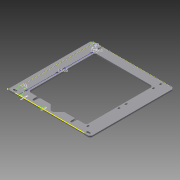
# Autodesk Inventor part: main_frame
Saved by Autodesk Inventor 2015 (Build 190159000, 159)
## iProperties
Created: 2014-12-25
Part Number: main_frame
Material: Generic
Document SubType Name: Modeling
Designer: X
Density: 1 g/cm^3
Appearance: Default
Author: X
Autodesk Inventor part; units mm, degrees
ref_plane "YZ Plane" through (0, 0, 0) normal (1, 0, 0) x (0, 1, 0)
ref_plane "XZ Plane" through (0, 0, 0) normal (0, 1, 0) x (-1, 0, 0)
ref_plane "XY Plane" through (0, 0, 0) normal (0, 0, 1) x (1, 0, 0)
sketch "Sketch1" plane through (0, 0, 0) normal (0, 0, 1) x (1, 0, 0)
  line L0 (7, 0) -> (363, 0)
  line L1 (370, 7) -> (370, 370)
  line L2 (363, 377) -> (7, 377)
  line L3 (0, 370) -> (0, 7)
  line L4 (7, 0) -> (0, 7)
  line L5 (-121.5053, 188.5) -> (511.4947, 188.5) construction
  line L6 (185, 402) -> (185, -38) construction
  line L7 (363, 0) -> (370, 7)
  line L8 (7, 377) -> (0, 370)
  line L9 (363, 377) -> (370, 370)
  point P0 (0, 0)
  point P1 (185, 377)
  point P2 (370, 188.5)
  dimension "height" = 370
  dimension "width" = 370
  dimension "Chamfer1" = 7
  dimension "Chamfer1ang" = 45
  constraints: 20 end point, 6 symmetric about line, 4 point on line, 2 horizontal, 2 midpoint, 2 parallel, 2 perpendicular
  measures "height" distance of L3.start point (0, 0)
  measures "width" distance between parallel lines of L3 L1
  measures "Chamfer1" distance of L0.start point (0, 0)
  measures "Chamfer1ang" angle of L0 L4
extrude "Extrusion1" add sketch "Sketch1" along normal blind 6
sketch "Sketch2" plane through (0, 0, 6) normal (0, 0, 1) x (1, 0, 0)
  line L0 (62, 337) -> (308, 337)
  line L1 (315, 330) -> (315, 45)
  line L2 (55, 45) -> (55, 330)
  line L3 (7, 377) -> (363, 377) projected
  line L4 (7, 0) -> (363, 0) projected
  line L5 (370, 370) -> (370, 7) projected
  line L6 (0, 370) -> (0, 7) projected
  line L7 (105, 34) -> (105, 18)
  line L8 (95, 18) -> (95, 34)
  line L9 (190, 13) -> (180, 13)
  line L10 (180, 13) -> (155, 38)
  line L11 (190, 13) -> (215, 38)
  line L12 (185, 422) -> (185, 5) construction
  arc A0 (95, 18) -> (105, 18) centre (100, 18) ccw
  line L13 (155, 38) -> (109, 38)
  line L14 (91, 38) -> (62, 38)
  line L15 (91, 38) -> (95, 34)
  line L16 (109, 38) -> (105, 34)
  line L17 (265, 34) -> (265, 18)
  line L18 (275, 18) -> (275, 34)
  arc A1 (265, 18) -> (275, 18) centre (270, 18) ccw
  line L19 (279, 38) -> (275, 34)
  line L20 (261, 38) -> (265, 34)
  line L21 (308, 38) -> (279, 38)
  line L22 (261, 38) -> (215, 38)
  line L23 (16, 187.5) -> (356, 187.5) construction
  line L24 (55, 45) -> (62, 38)
  line L25 (55, 330) -> (62, 337)
  line L26 (315, 45) -> (308, 38)
  line L27 (315, 330) -> (308, 337)
  point P0 (0, 0)
  point P1 (55, 38)
  point P2 (95, 38)
  point P3 (105, 38)
  point P4 (185, 337)
  point P5 (185, 13)
  point P6 (100, 13)
  point P7 (315, 187.5)
  dimension "top_dist" = 40
  dimension "Right_dist" = 55
  dimension "Left_dist" = 55
  dimension "width_triangle" = 10
  dimension "width_slot" = 10
  dimension "position_slot" = 40
  dimension "Height_triangle" = 25
  dimension "d30" = 25
  dimension "d31" = 4
  dimension "d32" = 4
  dimension "d33" = 4
  dimension "d34" = 4
  dimension "Bot_dist" = 38
  dimension "d36" = 7
  dimension "d37" = 7
  constraints: 48 end point, 13 symmetric about line, 9 point on line, 7 parallel, 5 point on circle, 4 collinear, 3 midpoint, 3 perpendicular, 2 centre point, 2 horizontal, 1 tangent, 2 other
  measures "top_dist" distance between parallel lines of L3 L0
  measures "Right_dist" distance between parallel lines of L5 L1
  measures "Left_dist" distance between parallel lines of L6 L2
  measures "width_triangle" distance of L9.start L9.end
  measures "width_slot" distance between parallel lines of L7 L8
  measures "position_slot" distance between parallel lines of L2 L8
  measures "Height_triangle" distance between parallel lines of L13 L9
  measures "d30" distance from line of L14 point (100, 13)
  measures "d31" distance of L14.start point (95, 38)
  measures "d32" distance of L8.end point (95, 38)
  measures "d33" distance of L13.end point (105, 38)
  measures "d34" distance of L7.start point (105, 38)
  measures "Bot_dist" distance between parallel lines of L4 L21
  measures "d36" distance of L2.start point (55, 38)
  measures "d37" distance of L14.end point (55, 38)
extrude "Extrusion2" cut sketch "Sketch2" against normal up to next
sketch "Sketch4" plane through (0, 0, 6) normal (0, 0, 1) x (1, 0, 0)
  line L0 (27, 0) -> (29, 2)
  line L1 (29, 2) -> (341, 2)
  line L2 (363, 0) -> (7, 0) projected
  line L3 (341, 2) -> (343, 0)
  line L4 (343, 0) -> (27, 0)
  line L5 (185, 2) -> (185, 0) construction
  point P0 (0, 0)
  dimension "d42" = 2
  dimension "d43" = 135
  dimension "d44" = 20
  dimension "d45" = 20
  constraints: 10 end point, 2 midpoint, 1 collinear, 1 parallel, 1 perpendicular, 1 point on line
  measures "d42" distance between parallel lines of L2 L1
  measures "d43" angle of L1 L0
  measures "d44" distance of L2.end L0.start
  measures "d45" distance of L2.start L3.end
extrude "Extrusion3" cut sketch "Sketch4" against normal through all
sketch "Sketch5" plane through (0, 0, 6) normal (0, 0, 1) x (1, 0, 0)
  line L0 (46.25, 377) -> (46.25, 2) construction
  line L1 (29, 2) -> (341, 2) construction
  line L2 (43, 358.743) -> (49.5, 358.743)
  line L3 (49.5, 358.743) -> (49.5, 367.743)
  line L4 (49.5, 367.743) -> (43, 367.743)
  line L5 (43, 367.743) -> (43, 358.743)
  line L6 (43, 358.743) -> (49.5, 367.743) construction
  line L7 (49.5, 358.743) -> (43, 367.743) construction
  line L8 (43, 326.443) -> (49.5, 326.443)
  line L9 (49.5, 326.443) -> (49.5, 335.443)
  line L10 (49.5, 335.443) -> (43, 335.443)
  line L11 (43, 335.443) -> (43, 326.443)
  line L12 (43, 326.443) -> (49.5, 335.443) construction
  line L13 (49.5, 326.443) -> (43, 335.443) construction
  line L14 (43, 203.65) -> (49.5, 203.65)
  line L15 (49.5, 203.65) -> (49.5, 212.65)
  line L16 (49.5, 212.65) -> (43, 212.65)
  line L17 (43, 212.65) -> (43, 203.65)
  line L18 (43, 203.65) -> (49.5, 212.65) construction
  line L19 (49.5, 203.65) -> (43, 212.65) construction
  line L20 (43, 171.35) -> (49.5, 171.35)
  line L21 (49.5, 171.35) -> (49.5, 180.35)
  line L22 (49.5, 180.35) -> (43, 180.35)
  line L23 (43, 180.35) -> (43, 171.35)
  line L24 (43, 171.35) -> (49.5, 180.35) construction
  line L25 (49.5, 171.35) -> (43, 180.35) construction
  line L26 (43, 32.15) -> (49.5, 32.15)
  line L27 (49.5, 32.15) -> (49.5, 41.15)
  line L28 (49.5, 41.15) -> (43, 41.15)
  line L29 (43, 41.15) -> (43, 32.15)
  line L30 (43, 32.15) -> (49.5, 41.15) construction
  line L31 (49.5, 32.15) -> (43, 41.15) construction
  line L32 (363, 377) -> (7, 377) projected
  line L33 (55, 45) -> (55, 330) projected
  line L34 (7, 377) -> (363, 377) construction
  line L35 (185, 377) -> (185, 2) construction
  line L36 (327, 358.743) -> (320.5, 358.743)
  line L37 (320.5, 358.743) -> (320.5, 367.743)
  line L38 (320.5, 367.743) -> (327, 367.743)
  line L39 (327, 367.743) -> (327, 358.743)
  line L40 (327, 326.443) -> (320.5, 326.443)
  line L41 (320.5, 326.443) -> (320.5, 335.443)
  line L42 (320.5, 335.443) -> (327, 335.443)
  line L43 (327, 335.443) -> (327, 326.443)
  line L44 (327, 203.65) -> (320.5, 203.65)
  line L45 (320.5, 203.65) -> (320.5, 212.65)
  line L46 (320.5, 212.65) -> (327, 212.65)
  line L47 (327, 212.65) -> (327, 203.65)
  line L48 (327, 171.35) -> (320.5, 171.35)
  line L49 (320.5, 171.35) -> (320.5, 180.35)
  line L50 (320.5, 180.35) -> (327, 180.35)
  line L51 (327, 180.35) -> (327, 171.35)
  line L52 (327, 32.15) -> (320.5, 32.15)
  line L53 (320.5, 32.15) -> (320.5, 41.15)
  line L54 (320.5, 41.15) -> (327, 41.15)
  line L55 (327, 41.15) -> (327, 32.15)
  point P0 (0, 0)
  point P1 (46.25, 363.243)
  point P2 (46.25, 330.943)
  point P3 (46.25, 208.15)
  point P4 (46.25, 175.85)
  point P5 (46.25, 36.65)
  dimension "d48" = 9
  dimension "d49" = 8.75
  dimension "d50" = 6.5
  dimension "d51" = 32.3
  dimension "d52" = 9.257
  dimension "d53" = 32.3
  dimension "d54" = 164.35
  dimension "d55" = 34.65
  constraints: 104 end point, 20 symmetric about line, 12 midpoint, 11 point on line, 10 parallel, 6 equal length, 5 horizontal, 5 perpendicular, 1 vertical
  measures "d48" distance of L4.end L2.start
  measures "d49" distance from line of point (46.25, 363.243) L33
  measures "d50" distance of L3.end L4.end
  measures "d51" distance of point (46.25, 330.943) point (46.25, 363.243)
  measures "d52" distance between parallel lines of L32 L4
  measures "d53" distance of point (46.25, 175.85) point (46.25, 208.15)
  measures "d54" distance between parallel lines of L32 L16
  measures "d55" distance from line of L1 point (46.25, 36.65)
extrude "Extrusion4" cut sketch "Sketch5" against normal through all
sketch "Sketch7" plane through (0, 0, 6) normal (0, 0, 1) x (1, 0, 0)
  circle A0 centre (16.026, 12.511) radius 4
  circle A1 centre (24.026, 12.511) radius 4
  line L0 (16.026, 16.511) -> (24.026, 16.511)
  line L1 (24.026, 8.511) -> (16.026, 8.511)
  line L2 (7, 0) -> (27, 0) projected
  line L3 (0, 370) -> (0, 7) projected
  line L4 (7, 377) -> (363, 377) construction
  line L5 (185, 377) -> (185, 2) construction
  line L6 (29, 2) -> (341, 2) construction
  circle A2 centre (353.974, 12.511) radius 4
  circle A3 centre (345.974, 12.511) radius 4
  line L7 (353.974, 16.511) -> (345.974, 16.511)
  line L8 (345.974, 8.511) -> (353.974, 8.511)
  point P0 (0, 0)
  dimension "d58" = 8
  dimension "d59" = 8
  dimension "d60" = 8.511
  dimension "d61" = 16.026
  constraints: 10 end point, 8 point on circle, 6 symmetric about line, 4 centre point, 3 tangent, 2 midpoint, 1 equal radius, 1 parallel, 2 other
  measures "d58" distance between parallel lines of L1 L0
  measures "d59" distance of L0.start L0.end
  measures "d60" distance between parallel lines of L2 L1
  measures "d61" distance from line of L3 A0.centre
extrude "Extrusion5" cut sketch "Sketch7" against normal through all
sketch "Sketch8" plane through (0, 0, 6) normal (0, 0, 1) x (1, 0, 0)
  line L0 (29, 2) -> (341, 2) projected
  line L1 (49.5, 358.743) -> (43, 358.743) construction
  line L2 (43, 358.743) -> (43, 367.743) construction
  line L3 (15.311, 367.093) -> (35.311, 367.093) construction
  line L4 (15.311, 40.093) -> (35.311, 40.093) construction
  line L5 (363, 377) -> (7, 377) construction
  line L6 (46.25, 377) -> (46.25, 2) construction
  line L7 (49.5, 203.65) -> (43, 203.65) construction
  line L8 (15.311, 40.093) -> (15.311, 367.093) construction
  point P0 (0, 0)
  point P1 (46.25, 347.093)
  point P2 (46.25, 192)
  point P3 (21, 22)
  point P4 (46.25, 24)
  point P5 (52, 6)
  point P6 (149, 6)
  dimension "d64" = 4
  dimension "d65" = 4
  dimension "d66" = 11.65
  dimension "d67" = 3.25
  dimension "d68" = 20
  dimension "d69" = 20
  dimension "d70" = 11.65
  dimension "d72" = 20
  constraints: 8 end point, 5 point on line, 3 parallel, 2 horizontal, 2 perpendicular
  measures "d64" distance from line of L0 point (149, 6)
  measures "d65" distance from line of L0 point (52, 6)
  measures "d66" distance from line of L1 point (46.25, 347.093)
  measures "d67" distance from line of L2 point (46.25, 347.093)
  measures "d68" distance of L3.end L3.start
  measures "d69" distance of L4.end L4.start
  measures "d70" distance from line of L7 point (46.25, 192)
  measures "d72" distance from line of point (46.25, 347.093) L3
equation "\"d32\" = d31"
equation "\"d34\" = d33"
equation "\"d37\" = d36"
body "Solid1"
